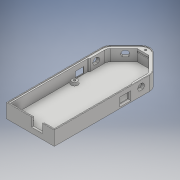
# Autodesk Inventor part: DynamicClampBottom
Saved by Autodesk Inventor 2017 (Build 210142000, 142)
## iProperties
Created: 2017-11-01
Part Number: DynamicClampBottom
Material: Generic
Document SubType Name: Modeling
Designer: andrew
Density: 1 g/cm^3
Appearance: Default
Author: andrew
Autodesk Inventor part; units mm, degrees
ref_plane "YZ Plane" through (0, 0, 0) normal (1, 0, 0) x (0, 1, 0)
ref_plane "XZ Plane" through (0, 0, 0) normal (0, 1, 0) x (-1, 0, 0)
ref_plane "XY Plane" through (0, 0, 0) normal (0, 0, 1) x (1, 0, 0)
sketch "Sketch1" plane through (0, 0, 0) normal (0, 0, 1) x (1, 0, 0)
  line L0 (0, 0) -> (66, 0) construction
  line L1 (66, 0) -> (66, 117) construction
  line L2 (0, 115.9019) -> (0, 0) construction
  line L3 (66, 115.9019) -> (66, 60.5) construction
  line L4 (65.9995, 1.253) -> (32.9995, 1.253) construction
  line L5 (32.9995, 1.253) -> (64.747, 1.253) construction
  line L6 (64.747, 1.253) -> (64.747, 48.238) construction
  line L7 (64.7475, 0) -> (64.7475, 1.253) construction
  line L8 (64.7475, 1.253) -> (60.9425, 1.253) construction
  line L9 (60.9425, 1.253) -> (60.9425, 5.058) construction
  line L10 (60.9425, 5.058) -> (64.7475, 5.058) construction
  line L11 (64.7475, 5.058) -> (64.7475, 1.253) construction
  circle A0 centre (60.9425, 5.058) radius 1.6 construction
  line L12 (65.9995, 95.223) -> (32.9995, 95.223) construction
  line L13 (32.9995, 95.223) -> (64.747, 95.223) construction
  line L14 (64.747, 95.223) -> (64.747, 48.238) construction
  line L15 (64.7475, 96.476) -> (64.7475, 95.223) construction
  line L16 (64.7475, 95.223) -> (60.9425, 95.223) construction
  line L17 (60.9425, 95.223) -> (60.9425, 91.418) construction
  line L18 (60.9425, 91.418) -> (64.7475, 91.418) construction
  line L19 (64.7475, 91.418) -> (64.7475, 95.223) construction
  circle A1 centre (60.9425, 91.418) radius 1.6 construction
  line L20 (-0.0005, 1.253) -> (32.9995, 1.253) construction
  line L21 (32.9995, 1.253) -> (1.252, 1.253) construction
  line L22 (1.252, 1.253) -> (1.252, 48.238) construction
  line L23 (1.2515, 0) -> (1.2515, 1.253) construction
  line L24 (1.2515, 1.253) -> (5.0565, 1.253) construction
  line L25 (5.0565, 1.253) -> (5.0565, 5.058) construction
  line L26 (5.0565, 5.058) -> (1.2515, 5.058) construction
  line L27 (1.2515, 5.058) -> (1.2515, 1.253) construction
  circle A2 centre (5.0565, 5.058) radius 1.6 construction
  line L28 (1.252, 95.223) -> (1.252, 48.238) construction
  line L29 (5.0565, 91.418) -> (1.2515, 91.418) construction
  circle A3 centre (5.0565, 91.418) radius 1.6 construction
  line L30 (1.2515, 91.418) -> (1.2515, 95.223) construction
  line L31 (1.2515, 95.223) -> (5.0565, 95.223) construction
  line L32 (5.0565, 95.223) -> (5.0565, 91.418) construction
  line L33 (1.2515, 96.476) -> (1.2515, 95.223) construction
  line L34 (-0.0005, 95.223) -> (32.9995, 95.223) construction
  line L35 (32.9995, 95.223) -> (1.252, 95.223) construction
  line L36 (32.9995, 95.223) -> (1.9995, 95.223) construction
  line L37 (1.9995, 95.223) -> (1.9995, 113.223) construction
  line L38 (1.9995, 113.223) -> (32.9995, 113.223) construction
  line L39 (32.9995, 113.223) -> (32.9995, 95.223) construction
  line L40 (63.9995, 95.223) -> (63.9995, 113.223) construction
  line L41 (63.9995, 113.223) -> (32.9995, 113.223) construction
  line L42 (41.8376, 166.5804) -> (24.1624, 166.5804)
  line L43 (3.8431, 146.2611) -> (24.1624, 166.5804)
  line L44 (41.8376, 166.5804) -> (62.1569, 146.2611)
  line L45 (64.8995, 149.8825) -> (42.1924, 172.5896)
  arc A4 (42.1924, 172.5896) -> (23.8076, 172.5896) centre (33, 163.3972) ccw
  line L46 (23.8076, 172.5896) -> (1.1005, 149.8825)
  line L47 (-3, -3) -> (69, -3) construction
  line L48 (69, -3) -> (69, 120) construction
  line L49 (-3, 117) -> (0, 117) construction
  arc A5 (1.252, 146.3272) -> (1.2515, 146.3253) centre (12.85, 143.2472) ccw
  arc A6 (0.85, 143.268) -> (0.85, 143.2472) centre (12.85, 143.2472) ccw
  arc A7 (4.3647, 151.7325) -> (4.35, 151.7177) centre (12.85, 143.2472) ccw
  line L50 (1.5, 118.5) -> (1.5, 140.6043)
  line L51 (69, 120) -> (69, 139.983)
  line L52 (64.5, 140.6043) -> (64.5, 118.5)
  line L53 (64.5, 117) -> (69, 117) construction
  line L54 (-3, -3) -> (69, -3)
  line L55 (69, 120) -> (69, -3)
  line L56 (66, 117) -> (66, 117)
  arc A8 (3.8431, 146.2611) -> (1.5, 140.6043) centre (9.5, 140.6043) ccw
  arc A9 (64.5, 140.6043) -> (62.1569, 146.2611) centre (56.5, 140.6043) ccw
  arc A10 (1.1005, 149.8825) -> (-3, 139.983) centre (11, 139.983) ccw
  arc A11 (69, 139.983) -> (64.8995, 149.8825) centre (55, 139.983) ccw
  arc A12 (0.75, 117.201) -> (1.5, 118.5) centre (0, 118.5) ccw
  arc A13 (0.75, 117.201) -> (0, 115.9019) centre (1.5, 115.9019) ccw
  line L57 (0, 115.9019) -> (0, 0)
  arc A14 (64.5, 118.5) -> (65.25, 117.201) centre (66, 118.5) ccw
  arc A15 (66, 115.9019) -> (65.25, 117.201) centre (64.5, 115.9019) ccw
  line L58 (66, 115.9019) -> (66, 0)
  line L59 (-3, -3) -> (-3, 139.983)
  dimension "d1" = 117
  dimension "d6" = 3.805
  dimension "d7" = 3.805
  dimension "d8" = 3.2
  dimension "d18" = 8
  dimension "d19" = 14
  dimension "d21" = 1.5
  constraints: 120 end point, 26 point on circle, 16 centre point, 15 tangent, 6 perpendicular, 6 point on line, 5 parallel, 4 coincident, 4 equal radius, 4 horizontal, 4 vertical, 3 collinear, 2 symmetric about line, 1 other
  measures "d1" distance of L1.end L0.end
  measures "d6" distance of L9.end L10.end
  measures "d7" distance of L8.end L9.end
  measures "d8" diameter of A0
  measures "d18" radius of A8
  measures "d19" radius of A10
  measures "d21" radius of A14
extrude "Extrusion1" add sketch "Sketch1" along normal blind 3 contours A8 L50 A5 L43 | L43 A5 L50 A8 | A11 L51 L55 L54 L59 A10 L46 A4 L45
sketch "Sketch2" plane through (0, 0, 3) normal (0, 0, 1) x (1, 0, 0)
  line L0 (0, 0) -> (66, 0) construction
  line L1 (66, 0) -> (66, 117) construction
  line L2 (0, 115.9019) -> (0, 0) construction
  line L3 (66, 115.9019) -> (66, 60.5) construction
  line L4 (65.9995, 1.253) -> (32.9995, 1.253) construction
  line L5 (32.9995, 1.253) -> (64.747, 1.253) construction
  line L6 (64.747, 1.253) -> (64.747, 48.238) construction
  line L7 (64.7475, 0) -> (64.7475, 1.253) construction
  line L8 (64.7475, 1.253) -> (60.9425, 1.253) construction
  line L9 (60.9425, 1.253) -> (60.9425, 5.058) construction
  line L10 (60.9425, 5.058) -> (64.7475, 5.058) construction
  line L11 (64.7475, 5.058) -> (64.7475, 1.253) construction
  circle A0 centre (60.9425, 5.058) radius 1.6 construction
  line L12 (64.747, 95.223) -> (64.747, 48.238) construction
  line L13 (60.9425, 91.418) -> (64.7475, 91.418) construction
  circle A1 centre (60.9425, 91.418) radius 1.6 construction
  line L14 (64.7475, 91.418) -> (64.7475, 95.223) construction
  line L15 (64.7475, 95.223) -> (60.9425, 95.223) construction
  line L16 (60.9425, 95.223) -> (60.9425, 91.418) construction
  line L17 (64.7475, 96.476) -> (64.7475, 95.223) construction
  line L18 (65.9995, 95.223) -> (32.9995, 95.223) construction
  line L19 (32.9995, 95.223) -> (64.747, 95.223) construction
  line L20 (32.9995, 95.223) -> (1.252, 95.223) construction
  line L21 (-0.0005, 95.223) -> (32.9995, 95.223) construction
  line L22 (1.2515, 91.418) -> (1.2515, 95.223) construction
  line L23 (5.0565, 91.418) -> (1.2515, 91.418) construction
  line L24 (5.0565, 95.223) -> (5.0565, 91.418) construction
  circle A2 centre (5.0565, 91.418) radius 1.6 construction
  line L25 (1.252, 95.223) -> (1.252, 48.238) construction
  line L26 (-0.0005, 1.253) -> (32.9995, 1.253) construction
  line L27 (32.9995, 1.253) -> (1.252, 1.253) construction
  line L28 (1.252, 1.253) -> (1.252, 48.238) construction
  line L29 (5.0565, 5.058) -> (1.2515, 5.058) construction
  circle A3 centre (5.0565, 5.058) radius 1.6 construction
  line L30 (5.0565, 1.253) -> (5.0565, 5.058) construction
  line L31 (1.2515, 5.058) -> (1.2515, 1.253) construction
  line L32 (1.2515, 1.253) -> (5.0565, 1.253) construction
  line L33 (1.2515, 0) -> (1.2515, 1.253) construction
  line L34 (1.2515, 95.223) -> (5.0565, 95.223) construction
  line L35 (1.2515, 96.476) -> (1.2515, 95.223) construction
  line L36 (32.9995, 95.223) -> (1.9995, 95.223) construction
  line L37 (1.9995, 95.223) -> (1.9995, 113.223) construction
  line L38 (1.9995, 113.223) -> (32.9995, 113.223) construction
  line L39 (32.9995, 113.223) -> (32.9995, 95.223) construction
  line L40 (63.9995, 113.223) -> (32.9995, 113.223) construction
  line L41 (63.9995, 95.223) -> (63.9995, 113.223) construction
  line L42 (3.8431, 146.2611) -> (24.1624, 166.5804)
  line L43 (23.8076, 172.5896) -> (1.1005, 149.8825)
  line L44 (41.8376, 166.5804) -> (24.1624, 166.5804)
  line L45 (41.8376, 166.5804) -> (62.1569, 146.2611)
  line L46 (64.8995, 149.8825) -> (42.1924, 172.5896)
  arc A4 (42.1924, 172.5896) -> (23.8076, 172.5896) centre (33, 163.3972) ccw
  line L47 (-3, -3) -> (69, -3) construction
  line L48 (69, -3) -> (69, 120) construction
  line L49 (-3, 117) -> (0, 117) construction
  arc A5 (1.252, 146.3272) -> (1.2515, 146.3253) centre (12.85, 143.2472) ccw
  arc A6 (0.85, 143.268) -> (0.85, 143.2472) centre (12.85, 143.2472) ccw
  arc A7 (4.3647, 151.7325) -> (4.35, 151.7177) centre (12.85, 143.2472) ccw
  line L50 (1.5, 118.5) -> (1.5, 140.6043)
  line L51 (69, 120) -> (69, 139.983)
  line L52 (64.5, 140.6043) -> (64.5, 118.5)
  line L53 (64.5, 117) -> (69, 117) construction
  line L54 (-3, -3) -> (69, -3)
  line L55 (69, 120) -> (69, -3)
  line L56 (66, 117) -> (66, 117)
  arc A8 (3.8431, 146.2611) -> (1.5, 140.6043) centre (9.5, 140.6043) ccw
  arc A9 (64.5, 140.6043) -> (62.1569, 146.2611) centre (56.5, 140.6043) ccw
  arc A10 (1.1005, 149.8825) -> (-3, 139.983) centre (11, 139.983) ccw
  arc A11 (69, 139.983) -> (64.8995, 149.8825) centre (55, 139.983) ccw
  arc A12 (0.75, 117.201) -> (1.5, 118.5) centre (0, 118.5) ccw
  arc A13 (0.75, 117.201) -> (0, 115.9019) centre (1.5, 115.9019) ccw
  line L57 (0, 115.9019) -> (0, 0)
  arc A14 (64.5, 118.5) -> (65.25, 117.201) centre (66, 118.5) ccw
  arc A15 (66, 115.9019) -> (65.25, 117.201) centre (64.5, 115.9019) ccw
  line L58 (66, 115.9019) -> (66, 0)
  line L59 (-3, -3) -> (-3, 139.983)
  line L60 (0, 0) -> (66, 0)
  dimension "d24" = 117
  dimension "d25" = 3.805
  dimension "d26" = 3.805
  dimension "d27" = 3.2
  dimension "d28" = 8
  dimension "d29" = 14
  dimension "d30" = 1.5
  constraints: 122 end point, 26 point on circle, 16 centre point, 15 tangent, 6 perpendicular, 6 point on line, 5 horizontal, 5 parallel, 4 coincident, 4 equal radius, 4 vertical, 3 collinear, 2 symmetric about line, 1 other
  measures "d24" distance of L1.end L0.end
  measures "d25" distance of L9.end L10.end
  measures "d26" distance of L8.end L9.end
  measures "d27" diameter of A0
  measures "d28" radius of A8
  measures "d29" radius of A10
  measures "d30" radius of A14
extrude "Extrusion2" add sketch "Sketch2" along normal blind 17.3 contours A8 L50 A5 L42 | A4 L46 A11 L51 L55 L54 L59 A10 L43 picked at (9.0553, 152.1739)
sketch "Sketch3" plane through (0, 0, 20.3) normal (0, 0, 1) x (1, 0, 0)
  arc A0 (0.75, 117.201) -> (0, 115.9019) centre (1.5, 115.9019) ccw projected
  arc A1 (0.75, 117.201) -> (1.5, 118.5) centre (0, 118.5) ccw projected
  line L0 (1.5, 118.5) -> (1.5, 140.6043) projected
  arc A2 (3.8431, 146.2611) -> (1.5, 140.6043) centre (9.5, 140.6043) ccw projected
  line L1 (3.8431, 146.2611) -> (24.1624, 166.5804) projected
  line L2 (24.1624, 166.5804) -> (41.8376, 166.5804) projected
  line L3 (41.8376, 166.5804) -> (62.1569, 146.2611) projected
  arc A3 (64.5, 140.6043) -> (62.1569, 146.2611) centre (56.5, 140.6043) ccw projected
  line L4 (64.5, 140.6043) -> (64.5, 118.5) projected
  arc A4 (64.5, 118.5) -> (65.25, 117.201) centre (66, 118.5) ccw projected
  arc A5 (66, 115.9019) -> (65.25, 117.201) centre (64.5, 115.9019) ccw projected
  line L5 (66, 115.9019) -> (66, 0) projected
  line L6 (66, 0) -> (0, 0) projected
  line L7 (0, 0) -> (0, 115.9019) projected
  arc A6 (42.1924, 172.5896) -> (23.8076, 172.5896) centre (33, 163.3972) ccw projected
  line L8 (23.8076, 172.5896) -> (1.1005, 149.8825) projected
  arc A7 (1.1005, 149.8825) -> (-3, 139.983) centre (11, 139.983) ccw projected
  line L9 (-3, 139.983) -> (-3, -3) projected
  line L10 (-3, -3) -> (69, -3) projected
  line L11 (69, -3) -> (69, 139.983) projected
  arc A8 (69, 139.983) -> (64.8995, 149.8825) centre (55, 139.983) ccw projected
  line L12 (64.8995, 149.8825) -> (42.1924, 172.5896) projected
  line L13 (-2, -2) -> (-2, 139.983)
  arc A9 (1.8076, 149.1754) -> (-2, 139.983) centre (11, 139.983) ccw
  line L14 (1.8076, 149.1754) -> (24.5147, 171.8825)
  arc A10 (41.4853, 171.8825) -> (24.5147, 171.8825) centre (33, 163.3972) ccw
  line L15 (41.4853, 171.8825) -> (64.1924, 149.1754)
  arc A11 (68, 139.983) -> (64.1924, 149.1754) centre (55, 139.983) ccw
  line L16 (68, 139.983) -> (68, -2)
  line L17 (68, -2) -> (-2, -2)
  dimension "d33" = 1
  constraints: 10 end point, 6 point on circle, 3 centre point, 7 other
  measures "d33" distance between parallel lines of L9 L13
extrude "Extrusion3" add sketch "Sketch3" along normal blind 1 contours L12 A8 L11 L10 L9 A7 L8 A6
sketch "Sketch5" plane through (-3, -3, 0) normal (-1, 0, 0) x (0, 0, 1)
  line L0 (0.01, 142.983) -> (21.3, 142.983)
  line L1 (8.12, 127.4284) -> (8.12, 133.5667)
  arc A0 (8.12, 127.4284) -> (8.12, 133.5667) centre (12.01, 130.4976) ccw
  line L2 (0, 0) -> (66, 0) construction
  line L3 (66, 0) -> (66, 117) construction
  line L4 (0, 115.9019) -> (0, 0) construction
  line L5 (66, 115.9019) -> (66, 60.5) construction
  line L6 (65.9995, 1.2535) -> (32.9995, 1.2535) construction
  line L7 (32.9995, 1.2535) -> (64.747, 1.2535) construction
  line L8 (64.747, 1.2535) -> (64.747, 48.2385) construction
  line L9 (64.7475, 0) -> (64.7475, 1.253) construction
  line L10 (64.7475, 1.253) -> (60.9425, 1.253) construction
  line L11 (60.9425, 1.253) -> (60.9425, 5.058) construction
  line L12 (60.9425, 5.058) -> (64.7475, 5.058) construction
  line L13 (64.7475, 5.058) -> (64.7475, 1.253) construction
  circle A1 centre (60.9425, 5.058) radius 1.6 construction
  line L14 (64.747, 95.2235) -> (64.747, 48.2385) construction
  line L15 (60.9425, 91.418) -> (64.7475, 91.418) construction
  circle A2 centre (60.9425, 91.418) radius 1.6 construction
  line L16 (64.7475, 91.418) -> (64.7475, 95.223) construction
  line L17 (64.7475, 95.223) -> (60.9425, 95.223) construction
  line L18 (60.9425, 95.223) -> (60.9425, 91.418) construction
  line L19 (64.7475, 96.476) -> (64.7475, 95.223) construction
  line L20 (65.9995, 95.2235) -> (32.9995, 95.2235) construction
  line L21 (32.9995, 95.2235) -> (64.747, 95.2235) construction
  line L22 (32.9995, 95.2235) -> (1.252, 95.2235) construction
  line L23 (-0.0005, 95.2235) -> (32.9995, 95.2235) construction
  line L24 (1.2515, 91.418) -> (1.2515, 95.223) construction
  line L25 (5.0565, 91.418) -> (1.2515, 91.418) construction
  line L26 (5.0565, 95.223) -> (5.0565, 91.418) construction
  circle A3 centre (5.0565, 91.418) radius 1.6 construction
  line L27 (1.252, 95.2235) -> (1.252, 48.2385) construction
  line L28 (-0.0005, 1.2535) -> (32.9995, 1.2535) construction
  line L29 (32.9995, 1.2535) -> (1.252, 1.2535) construction
  line L30 (1.252, 1.2535) -> (1.252, 48.2385) construction
  line L31 (5.0565, 5.058) -> (1.2515, 5.058) construction
  circle A4 centre (5.0565, 5.058) radius 1.6 construction
  line L32 (5.0565, 1.253) -> (5.0565, 5.058) construction
  line L33 (1.2515, 5.058) -> (1.2515, 1.253) construction
  line L34 (1.2515, 1.253) -> (5.0565, 1.253) construction
  line L35 (1.2515, 0) -> (1.2515, 1.253) construction
  line L36 (1.2515, 95.223) -> (5.0565, 95.223) construction
  line L37 (1.2515, 96.476) -> (1.2515, 95.223) construction
  line L38 (32.9995, 95.2235) -> (1.9995, 95.2235) construction
  line L39 (1.9995, 95.2235) -> (1.9995, 113.2235) construction
  line L40 (32.9995, 113.2235) -> (32.9995, 95.2235) construction
  line L41 (63.9995, 113.2235) -> (32.9995, 113.2235) construction
  line L42 (63.9995, 95.2235) -> (63.9995, 113.2235) construction
  line L43 (3.8431, 146.2611) -> (24.1624, 166.5804)
  line L44 (23.8076, 172.5896) -> (1.1005, 149.8825)
  line L45 (41.8376, 166.5804) -> (24.1624, 166.5804)
  line L46 (41.8376, 166.5804) -> (62.1569, 146.2611)
  line L47 (64.8995, 149.8825) -> (42.1924, 172.5896)
  arc A5 (42.1924, 172.5896) -> (23.8076, 172.5896) centre (33, 163.3972) ccw
  line L48 (-3, -3) -> (69, -3) construction
  line L49 (69, -3) -> (69, 120) construction
  line L50 (-3, 117) -> (0, 117) construction
  arc A6 (1.252, 146.3272) -> (1.2515, 146.3253) centre (12.85, 143.2472) ccw
  arc A7 (0.85, 143.268) -> (0.85, 143.2472) centre (12.85, 143.2472) ccw
  arc A8 (4.3647, 151.7325) -> (4.35, 151.7177) centre (12.85, 143.2472) ccw
  line L51 (1.5, 118.5) -> (1.5, 140.6043)
  line L52 (69, 120) -> (69, 139.983)
  line L53 (64.5, 140.6043) -> (64.5, 118.5)
  line L54 (64.5, 117) -> (69, 117) construction
  line L55 (-3, -3) -> (69, -3)
  line L56 (69, 120) -> (69, -3)
  line L57 (66, 117) -> (66, 117)
  arc A9 (3.8431, 146.2611) -> (1.5, 140.6043) centre (9.5, 140.6043) ccw
  arc A10 (64.5, 140.6043) -> (62.1569, 146.2611) centre (56.5, 140.6043) ccw
  arc A11 (1.1005, 149.8825) -> (-3, 139.983) centre (11, 139.983) ccw
  arc A12 (69, 139.983) -> (64.8995, 149.8825) centre (55, 139.983) ccw
  arc A13 (0.75, 117.201) -> (1.5, 118.5) centre (0, 118.5) ccw
  arc A14 (0.75, 117.201) -> (0, 115.9019) centre (1.5, 115.9019) ccw
  line L58 (0, 115.9019) -> (0, 0)
  arc A15 (64.5, 118.5) -> (65.25, 117.201) centre (66, 118.5) ccw
  arc A16 (66, 115.9019) -> (65.25, 117.201) centre (64.5, 115.9019) ccw
  line L59 (66, 115.9019) -> (66, 0)
  line L60 (-3, -3) -> (-3, 139.983)
  line L61 (3, 120.201) -> (3, 118.9019) projected
  line L62 (3, 118.9019) -> (3, 3) projected
  line L63 (3, 3) -> (3, 118.9019) projected
  line L64 (3, 118.9019) -> (3, 120.201) projected
  line L65 (3, 120.201) -> (3, 121.5) projected
  line L66 (3, 121.5) -> (3, 143.6043) projected
  line L67 (3, 143.6043) -> (3, 149.2611) projected
  line L68 (3, 149.2611) -> (3, 169.5804) projected
  line L69 (3, 169.5804) -> (3, 149.2611) projected
  line L70 (3, 149.2611) -> (3, 143.6043) projected
  line L71 (3, 143.6043) -> (3, 121.5) projected
  line L72 (3, 121.5) -> (3, 120.201) projected
  line L73 (3, 3) -> (3, 118.9019) projected
  line L74 (3, 113.223) -> (3, 95.2235)
  line L75 (3, 107.0625) -> (4, 107.0625)
  line L76 (4, 113.3125) -> (13, 113.3125)
  line L77 (13, 113.3125) -> (13, 100.8125)
  line L78 (13, 100.8125) -> (4, 100.8125)
  line L79 (4, 100.8125) -> (4, 113.3125)
  line L80 (4, 107.0625) -> (8.5, 107.0625) construction
  line L81 (8.5, 107.0625) -> (8.5, 100.8125) construction
  line L82 (8.5, 100.8125) -> (4, 100.8125) construction
  line L83 (4, 100.8125) -> (4, 107.0625) construction
  line L84 (3, 118.9019) -> (20.3, 118.9019) projected
  line L85 (20.5496, 124.5804) -> (20.5496, 95.2235)
  line L86 (20.5496, 109.9019) -> (8.5, 109.9019)
  line L87 (20.5496, 109.9019) -> (32.5992, 109.9019) construction
  point P0 (0, 3)
  point P1 (6.7, 40.8872)
  point P2 (3, 98.418)
  point P3 (3, 90.418)
  point P4 (3, 12.058)
  point P5 (3, 4.058)
  point P6 (3, 12.058)
  point P7 (3, 4.058)
  point P8 (3, 98.418)
  point P9 (3, 90.418)
  dimension "d63" = 117
  dimension "d64" = 3.805
  dimension "d65" = 3.805
  dimension "d66" = 3.2
  dimension "d67" = 8
  dimension "d68" = 14
  dimension "d69" = 1.5
  dimension "d70" = 1
  dimension "d71" = 9
  dimension "d72" = 12.5
  dimension "d87" = 5.589
  dimension "d88" = 180
  constraints: 148 end point, 28 point on circle, 17 centre point, 15 tangent, 9 perpendicular, 8 horizontal, 8 parallel, 8 point on line, 4 coincident, 4 collinear, 4 equal radius, 4 vertical, 3 midpoint, 2 symmetric about line, 4 other
  measures "d63" distance of L3.end L2.end
  measures "d64" distance of L11.end L12.end
  measures "d65" distance of L10.end L11.end
  measures "d66" diameter of A1
  measures "d67" radius of A9
  measures "d68" radius of A11
  measures "d69" radius of A15
  measures "d70" distance of L75.start L75.end
  measures "d71" distance of L77.end L78.end
  measures "d72" distance of L76.end L77.end
  measures "d87" distance between parallel lines of L38 L78
  measures "d88" angle of L86 L87
extrude "Extrusion5" cut sketch "Sketch5" against normal blind 100 contours A6 A0 L1 | L1 A0 A6 | L76 L77 L78 L79
sketch "Sketch4" plane through (0, 0, 3) normal (0, 0, 1) x (1, 0, 0)
  line L0 (0, 0) -> (66, 0) construction
  line L1 (66, 0) -> (66, 117) construction
  line L2 (0, 115.9019) -> (0, 0) construction
  line L3 (66, 115.9019) -> (66, 60.5) construction
  line L4 (65.9995, 1.253) -> (32.9995, 1.253) construction
  line L5 (32.9995, 1.253) -> (64.747, 1.253) construction
  line L6 (64.747, 1.253) -> (64.747, 48.238) construction
  line L7 (64.7475, 0) -> (64.7475, 1.253) construction
  line L8 (64.7475, 1.253) -> (60.9425, 1.253) construction
  line L9 (60.9425, 1.253) -> (60.9425, 5.058) construction
  line L10 (60.9425, 5.058) -> (64.7475, 5.058) construction
  line L11 (64.7475, 5.058) -> (64.7475, 1.253) construction
  circle A0 centre (60.9425, 5.058) radius 1.6
  line L12 (64.747, 95.223) -> (64.747, 48.238) construction
  line L13 (60.9425, 91.418) -> (64.7475, 91.418) construction
  circle A1 centre (60.9425, 91.418) radius 1.6
  line L14 (64.7475, 91.418) -> (64.7475, 95.223) construction
  line L15 (64.7475, 95.223) -> (60.9425, 95.223) construction
  line L16 (60.9425, 95.223) -> (60.9425, 91.418) construction
  line L17 (64.7475, 96.476) -> (64.7475, 95.223) construction
  line L18 (65.9995, 95.223) -> (32.9995, 95.223) construction
  line L19 (32.9995, 95.223) -> (64.747, 95.223) construction
  line L20 (32.9995, 95.223) -> (1.252, 95.223) construction
  line L21 (-0.0005, 95.223) -> (32.9995, 95.223) construction
  line L22 (1.2515, 91.418) -> (1.2515, 95.223) construction
  line L23 (5.0565, 91.418) -> (1.2515, 91.418) construction
  line L24 (5.0565, 95.223) -> (5.0565, 91.418) construction
  circle A2 centre (5.0565, 91.418) radius 1.6
  line L25 (1.252, 95.223) -> (1.252, 48.238) construction
  line L26 (-0.0005, 1.253) -> (32.9995, 1.253) construction
  line L27 (32.9995, 1.253) -> (1.252, 1.253) construction
  line L28 (1.252, 1.253) -> (1.252, 48.238) construction
  line L29 (5.0565, 5.058) -> (1.2515, 5.058) construction
  circle A3 centre (5.0565, 5.058) radius 1.6
  line L30 (5.0565, 1.253) -> (5.0565, 5.058) construction
  line L31 (1.2515, 5.058) -> (1.2515, 1.253) construction
  line L32 (1.2515, 1.253) -> (5.0565, 1.253) construction
  line L33 (1.2515, 0) -> (1.2515, 1.253) construction
  line L34 (1.2515, 95.223) -> (5.0565, 95.223) construction
  line L35 (1.2515, 96.476) -> (1.2515, 95.223) construction
  line L36 (32.9995, 95.223) -> (1.9995, 95.223) construction
  line L37 (1.9995, 95.223) -> (1.9995, 113.223) construction
  line L38 (1.9995, 113.223) -> (32.9995, 113.223) construction
  line L39 (32.9995, 113.223) -> (32.9995, 95.223) construction
  line L40 (63.9995, 113.223) -> (32.9995, 113.223) construction
  line L41 (63.9995, 95.223) -> (63.9995, 113.223) construction
  line L42 (3.8431, 146.2611) -> (24.1624, 166.5804)
  line L43 (23.8076, 172.5896) -> (1.1005, 149.8825)
  line L44 (41.8376, 166.5804) -> (24.1624, 166.5804)
  line L45 (41.8376, 166.5804) -> (62.1569, 146.2611)
  line L46 (64.8995, 149.8825) -> (42.1924, 172.5896)
  arc A4 (42.1924, 172.5896) -> (23.8076, 172.5896) centre (33, 163.3972) ccw
  line L47 (-3, -3) -> (69, -3) construction
  line L48 (69, -3) -> (69, 120) construction
  line L49 (-3, 117) -> (0, 117) construction
  arc A5 (1.252, 146.3272) -> (1.2515, 146.3253) centre (12.85, 143.2472) ccw
  arc A6 (0.85, 143.268) -> (0.85, 143.2472) centre (12.85, 143.2472) ccw
  arc A7 (4.3647, 151.7325) -> (4.35, 151.7177) centre (12.85, 143.2472) ccw
  line L50 (1.5, 118.5) -> (1.5, 140.6043)
  line L51 (69, 120) -> (69, 139.983)
  line L52 (64.5, 140.6043) -> (64.5, 118.5)
  line L53 (64.5, 117) -> (69, 117) construction
  line L54 (-3, -3) -> (69, -3)
  line L55 (69, 120) -> (69, -3)
  line L56 (66, 117) -> (66, 117)
  arc A8 (3.8431, 146.2611) -> (1.5, 140.6043) centre (9.5, 140.6043) ccw
  arc A9 (64.5, 140.6043) -> (62.1569, 146.2611) centre (56.5, 140.6043) ccw
  arc A10 (1.1005, 149.8825) -> (-3, 139.983) centre (11, 139.983) ccw
  arc A11 (69, 139.983) -> (64.8995, 149.8825) centre (55, 139.983) ccw
  arc A12 (0.75, 117.201) -> (1.5, 118.5) centre (0, 118.5) ccw
  arc A13 (0.75, 117.201) -> (0, 115.9019) centre (1.5, 115.9019) ccw
  line L57 (0, 115.9019) -> (0, 0)
  arc A14 (64.5, 118.5) -> (65.25, 117.201) centre (66, 118.5) ccw
  arc A15 (66, 115.9019) -> (65.25, 117.201) centre (64.5, 115.9019) ccw
  line L58 (66, 115.9019) -> (66, 0)
  line L59 (-3, -3) -> (-3, 139.983)
  circle A16 centre (5.0565, 5.058) radius 4
  circle A17 centre (60.9425, 5.058) radius 4
  circle A18 centre (5.0565, 91.418) radius 4
  circle A19 centre (60.9425, 91.418) radius 4
  dimension "d36" = 117
  dimension "d37" = 3.805
  dimension "d38" = 3.805
  dimension "d39" = 3.2
  dimension "d40" = 8
  dimension "d41" = 14
  dimension "d42" = 1.5
  dimension "d43" = 8
  dimension "d44" = 8
  dimension "d45" = 8
  dimension "d46" = 8
  constraints: 120 end point, 26 point on circle, 20 centre point, 15 tangent, 8 coincident, 6 perpendicular, 6 point on line, 5 parallel, 4 equal radius, 4 horizontal, 4 vertical, 3 collinear, 2 symmetric about line, 1 other
  measures "d36" distance of L1.end L0.end
  measures "d37" distance of L9.end L10.end
  measures "d38" distance of L8.end L9.end
  measures "d39" diameter of A0
  measures "d40" radius of A8
  measures "d41" radius of A10
  measures "d42" radius of A14
  measures "d43" diameter of A16
  measures "d44" diameter of A17
  measures "d45" diameter of A18
  measures "d46" diameter of A19
extrude "Extrusion4" add sketch "Sketch4" along normal blind 4 contours A16 | A17 | A18 | A19
sketch "Sketch6" plane through (1.1005, 149.8825, 21.3) normal (-0.7071068, 0.7071068, 0) x (0.7071068, 0.7071068, 0)
  line L0 (12.3053, 11.8312) -> (18.6412, 11.8312)
  arc A0 (12.3053, 11.8312) -> (18.6412, 11.8312) centre (15.4732, 8.0212) ccw
  line L1 (0, 21.29) -> (0, 0)
  line L2 (28.4964, 0) -> (0, 0)
  line L3 (28.4964, 21.29) -> (28.4964, 0)
  line L4 (0, 21.29) -> (28.4964, 21.29)
  point P0 (-106.7611, 21.3)
  constraints: 10 end point, 2 point on circle, 1 centre point
extrude "Extrusion6" cut sketch "Sketch6" against normal blind 10 contours L0 A0
sketch "Sketch7" plane through (42.1924, 172.5896, 21.3) normal (0.7071068, 0.7071068, 0) x (0, 0, -1)
  line L0 (11.8312, -15.9216) -> (11.8312, -22.2575)
  arc A0 (11.8312, -15.9216) -> (11.8312, -22.2575) centre (8.0212, -19.0895) ccw
  line L1 (21.29, -3.6163) -> (0, -3.6163)
  line L2 (0, -32.1127) -> (0, -3.6163)
  line L3 (21.29, -32.1127) -> (0, -32.1127)
  line L4 (21.29, -3.6163) -> (21.29, -32.1127)
  point P0 (21.3, -92.2047)
  constraints: 10 end point, 2 point on circle, 1 centre point
extrude "Extrusion7" cut sketch "Sketch7" against normal blind 10 contours L0 A0
chamfer "Chamfer5" distance 2 angle 45 4 edges at (-3, 110.3125, 8.5) (-3, 104.0625, 4) (-3, 97.8125, 8.5) (-3, 104.0625, 13)
chamfer "Chamfer6" distance 2 angle 45 4 edges at (69, 104.0625, 4) (69, 97.8125, 8.5) (69, 104.0625, 13) (69, 110.3125, 8.5)
sketch "Sketch10" plane through (0, 0, 7) normal (0, 0, 1) x (1, 0, 0)
  circle A0 centre (5.0565, 5.058) radius 1.6 projected
  circle A1 centre (5.0565, 91.418) radius 1.6 projected
  circle A2 centre (60.9425, 5.058) radius 1.6 projected
  circle A3 centre (60.9425, 91.418) radius 1.6 projected
  point P0 (0, 0)
extrude "Extrusion8" cut sketch "Sketch10" against normal blind 6
sketch "Sketch11" plane through (-3, -3, 0) normal (0, -1, 0) x (1, 0, 0)
  line L0 (4.0565, 3) -> (12.0565, 3) projected
  line L1 (6.4565, 7) -> (9.6565, 7) projected
  line L2 (12.0565, 7) -> (4.0565, 7) projected
  line L3 (62.3425, 7) -> (65.5425, 7) construction
  line L4 (67.9425, 7) -> (59.9425, 7) construction
  line L5 (4.0565, 7) -> (35.9995, 7) construction
  line L6 (4.1005, 0) -> (4.1005, 21.3) projected
  line L7 (35.9995, 7) -> (35.9995, 8) construction
  line L8 (35.9995, 8) -> (35.9995, 19) construction
  line L9 (53.9995, 19) -> (55.9995, 19) construction
  line L10 (55.9995, 8) -> (55.9995, 7) construction
  line L11 (35.9995, 8) -> (55.9995, 8) construction
  line L12 (35.9995, 8) -> (37.9995, 8) construction
  line L13 (37.9995, 8) -> (37.9995, 19) construction
  line L14 (55.9995, 8) -> (53.9995, 8) construction
  line L15 (53.9995, 8) -> (53.9995, 19) construction
  line L16 (37.9995, 19) -> (37.9995, 24.5991) construction
  line L17 (37.9995, 24.5991) -> (53.9995, 24.5991) construction
  line L18 (53.9995, 24.5991) -> (53.9995, 19) construction
  line L19 (37.9995, 24.5991) -> (53.9995, 24.5991)
  line L20 (53.9995, 24.5991) -> (53.9995, 8)
  line L21 (53.9995, 8) -> (37.9995, 8)
  line L22 (37.9995, 8) -> (37.9995, 24.5991)
  point P0 (3, 0)
  dimension "d89" = 1
  dimension "d90" = 11
  dimension "d91" = 20
  dimension "d102" = 2
  dimension "d103" = 2
  constraints: 34 end point, 9 perpendicular, 3 vertical, 2 parallel, 2 point on line, 1 horizontal
  measures "d89" distance of L5.end L7.end
  measures "d90" distance of L7.end L8.end
  measures "d91" distance of L8.end L9.end
  measures "d102" distance of L7.end L12.end
  measures "d103" distance of L10.start L14.end
extrude "Extrusion9" cut sketch "Sketch11" against normal blind 6
sketch "Sketch12" plane through (0, 0, 3) normal (0, 1, 0) x (1, 0, 0)
  line L0 (0, -6.3) -> (0, -18.3) construction
  line L1 (0, -17.3) -> (15.9851, -17.3) construction
  line L2 (7.9925, -17.3) -> (7.9925, -14.3) construction
  line L3 (7.9925, -14.3) -> (15.9851, -14.3) construction
  line L4 (15.9851, -12.3) -> (0, -12.3) construction
  line L5 (15.9851, -14.3) -> (0, -14.3) construction
  line L6 (0, -14.3) -> (0, -12.3) construction
  line L7 (0, -12.3) -> (15.9851, -12.3) construction
  line L8 (1.8076, -17.3) -> (-2, -17.3) construction
  line L9 (-2, -17.3) -> (34.9995, -17.3) construction
  line L10 (68, -17.3) -> (64.1924, -17.3) construction
  line L11 (64.1924, -17.3) -> (41.4853, -17.3) construction
  line L12 (41.4853, -17.3) -> (24.5147, -17.3) construction
  line L13 (24.5147, -17.3) -> (1.8076, -17.3) construction
  line L14 (0, -17.3) -> (0.75, -17.3) construction
  line L15 (0.75, -17.3) -> (1.5, -17.3) construction
  line L16 (1.5, -17.3) -> (3.8431, -17.3) construction
  line L17 (3.8431, -17.3) -> (24.1624, -17.3) construction
  line L18 (24.1624, -17.3) -> (41.8376, -17.3) construction
  line L19 (41.8376, -17.3) -> (62.1569, -17.3) construction
  line L20 (62.1569, -17.3) -> (64.5, -17.3) construction
  line L21 (64.5, -17.3) -> (65.25, -17.3) construction
  line L22 (65.25, -17.3) -> (66, -17.3) construction
  line L23 (66, -17.3) -> (50.9995, -17.3) construction
  line L24 (69, 3) -> (-3, 3) construction
  line L25 (69, 3) -> (69, -18.3) construction
  line L26 (-3, -18.3) -> (34.9995, -18.3) construction
  line L27 (-3, 3) -> (-3, -18.3) construction
  line L28 (66, -1) -> (66, -10) construction
  line L29 (66, -10) -> (66, -1) construction
  line L30 (66, 0) -> (66, -17.3) construction
  line L31 (66, 0) -> (66, -17.3) construction
  line L32 (66, 0) -> (66, -17.3) construction
  line L33 (15.9851, -12.3) -> (66, -12.3) construction
  line L34 (66, -12.3) -> (66, -14.3) construction
  line L35 (66, -14.3) -> (15.9851, -14.3) construction
  line L36 (0, -14.3) -> (66, -14.3)
  line L37 (66, -14.3) -> (66, -12.3)
  line L38 (66, -12.3) -> (0, -12.3)
  line L39 (0, -12.3) -> (0, -14.3)
  line L40 (34.9995, -5) -> (34.9995, -18.3) projected
  line L41 (50.9995, -18.3) -> (69, -18.3) projected
  line L42 (50.9995, -18.3) -> (50.9995, -5) projected
  line L43 (50.9995, -5) -> (34.9995, -5) projected
  line L44 (34.9995, -17.3) -> (0, -17.3) projected
  line L45 (50.9995, -17.3) -> (68, -17.3) projected
  point P0 (0, 3)
  dimension "d94" = 3
  dimension "d95" = 2
  constraints: 30 end point, 4 parallel, 4 perpendicular, 3 horizontal, 2 midpoint, 1 vertical, 2 other
  measures "d94" distance of L2.start L2.end
  measures "d95" distance of L3.end L4.start
extrude "Extrusion10" cut sketch "Sketch12" against normal blind 1 contours L39 L38 L40 L36 | L40 L38 L42 L36 | L42 L38 L37 L36
sketch "Sketch13" plane through (0, 0, 20.3) normal (0, 0, 1) x (1, 0, 0)
  circle A0 centre (-63.0458, -19.0499) radius 1.6
  circle A1 centre (-63.0458, -19.0499) radius 1.6
  line L0 (-71.8833, -22.7667) -> (-54.2082, -22.7667)
  line L1 (-54.2082, -22.7667) -> (-36.8854, -40.0895)
  line L2 (-34.4105, -37.6146) -> (-54.5605, -17.4646)
  arc A2 (-54.5605, -17.4646) -> (-71.5311, -17.4646) centre (-63.0458, -25.9499) ccw
  line L3 (-71.5311, -17.4646) -> (-91.6811, -37.6146)
  line L4 (-89.2062, -40.0895) -> (-71.8833, -22.7667)
  circle A3 centre (-63.0458, -19.0499) radius 1.6
  circle A4 centre (-63.0458, -19.0499) radius 1.6
  line L5 (-71.8833, -22.7667) -> (-54.2082, -22.7667)
  line L6 (-54.2082, -22.7667) -> (-36.8854, -40.0895)
  line L7 (-34.4105, -37.6146) -> (-54.5605, -17.4646)
  arc A5 (-54.5605, -17.4646) -> (-71.5311, -17.4646) centre (-63.0458, -25.9499) ccw
  line L8 (-71.5311, -17.4646) -> (-91.6811, -37.6146)
  line L9 (-89.2062, -40.0895) -> (-71.8833, -22.7667)
  arc A6 (42.1924, 172.5896) -> (23.8076, 172.5896) centre (33, 163.3972) ccw projected
  circle A7 centre (32.2929, 171.0043) radius 1.6
  point P0 (0, 0)
  constraints: 20 end point, 7 centre point, 4 point on circle
extrude "Extrusion11" cut sketch "Sketch13" against normal blind 12 contours A7
sketch "Sketch14" plane through (24.1624, 166.5804, 3) normal (0, -1, 0) x (1, 0, 0)
  line L0 (17.6751, 0) -> (0, 0) construction
  line L1 (17.6751, 0) -> (17.6751, 17.3) construction
  line L2 (0, 17.3) -> (17.6751, 17.3) construction
  line L3 (0, 0) -> (0, 17.3) construction
  line L4 (41.8376, 14.3) -> (-24.1624, 14.3) construction
  line L5 (-24.1624, 12.3) -> (10.8371, 12.3) construction
  line L6 (-24.1624, 12.3) -> (10.8371, 12.3) construction
  line L7 (0, 12.3) -> (17.6751, 12.3) construction
  line L8 (17.6751, 12.3) -> (17.6751, 14.3) construction
  line L9 (17.6751, 14.3) -> (0, 14.3) construction
  line L10 (0, 14.3) -> (0, 12.3) construction
  line L11 (0, 12.3) -> (17.6751, 12.3)
  line L12 (17.6751, 12.3) -> (17.6751, 14.3)
  line L13 (17.6751, 14.3) -> (0, 14.3)
  line L14 (0, 14.3) -> (0, 12.3)
  point P0 (-24.1624, -3)
  point P1 (8.8371, 12.3)
  constraints: 16 end point, 4 parallel, 4 point on line, 2 horizontal, 2 perpendicular
extrude "Extrusion12" cut sketch "Sketch14" against normal blind 1
chamfer "Chamfer7" distance 1 distance2 4 1 edges at (1.0565, 5.058, 3) measured on face at (24.4426, 34.942, 3)
chamfer "Chamfer8" distance 1 distance2 4 1 edges at (56.9425, 5.058, 3) measured on face at (24.6319, 61.8083, 3)
chamfer "Chamfer9" distance 1 distance2 4 1 edges at (56.9425, 91.418, 3) measured on face at (24.6319, 61.8083, 3)
chamfer "Chamfer10" distance 1 distance2 4 1 edges at (1.0565, 91.418, 3) measured on face at (24.4426, 61.534, 3)
body "Solid1"
